Autodesk Inventor part; units mm, degrees
(part 2 of 2)
  line L450 (57.93, 7.062) -> (57.93, 1.062)
  line L451 (63.93, 7.062) -> (57.93, 7.062)
  line L452 (63.93, 1.062) -> (63.93, 7.062)
  line L453 (63.43, 6.562) -> (63.43, 1.562)
  line L454 (63.43, 1.562) -> (58.43, 1.562)
  line L455 (58.43, 1.562) -> (58.43, 6.562)
  line L456 (58.43, 6.562) -> (63.43, 6.562)
  line L457 (57.93, 9.186) -> (63.93, 9.186)
  line L458 (57.93, 15.186) -> (57.93, 9.186)
  line L459 (63.93, 15.186) -> (57.93, 15.186)
  line L460 (63.93, 9.186) -> (63.93, 15.186)
  line L461 (63.43, 14.686) -> (63.43, 9.686)
  line L462 (63.43, 9.686) -> (58.43, 9.686)
  line L463 (58.43, 9.686) -> (58.43, 14.686)
  line L464 (58.43, 14.686) -> (63.43, 14.686)
  line L465 (57.93, 17.31) -> (63.93, 17.31)
  line L466 (57.93, 23.31) -> (57.93, 17.31)
  line L467 (63.93, 23.31) -> (57.93, 23.31)
  line L468 (63.93, 17.31) -> (63.93, 23.31)
  line L469 (63.43, 22.81) -> (63.43, 17.81)
  line L470 (63.43, 17.81) -> (58.43, 17.81)
  line L471 (58.43, 17.81) -> (58.43, 22.81)
  line L472 (58.43, 22.81) -> (63.43, 22.81)
  line L473 (57.93, 25.434) -> (63.93, 25.434)
  line L474 (57.93, 31.434) -> (57.93, 25.434)
  line L475 (63.93, 31.434) -> (57.93, 31.434)
  line L476 (63.93, 25.434) -> (63.93, 31.434)
  line L477 (63.43, 30.934) -> (63.43, 25.934)
  line L478 (63.43, 25.934) -> (58.43, 25.934)
  line L479 (58.43, 25.934) -> (58.43, 30.934)
  line L480 (58.43, 30.934) -> (63.43, 30.934)
  line L481 (57.93, 33.558) -> (63.93, 33.558)
  line L482 (57.93, 39.558) -> (57.93, 33.558)
  line L483 (63.93, 39.558) -> (57.93, 39.558)
  line L484 (63.93, 33.558) -> (63.93, 39.558)
  line L485 (63.43, 39.058) -> (63.43, 34.058)
  line L486 (63.43, 34.058) -> (58.43, 34.058)
  line L487 (58.43, 34.058) -> (58.43, 39.058)
  line L488 (58.43, 39.058) -> (63.43, 39.058)
  line L489 (57.93, 41.682) -> (63.93, 41.682)
  line L490 (57.93, 47.682) -> (57.93, 41.682)
  line L491 (63.93, 47.682) -> (57.93, 47.682)
  line L492 (63.93, 41.682) -> (63.93, 47.682)
  line L493 (63.43, 47.182) -> (63.43, 42.182)
  line L494 (63.43, 42.182) -> (58.43, 42.182)
  line L495 (58.43, 42.182) -> (58.43, 47.182)
  line L496 (58.43, 47.182) -> (63.43, 47.182)
  line L497 (57.93, 49.806) -> (63.93, 49.806)
  line L498 (57.93, 55.806) -> (57.93, 49.806)
  line L499 (63.93, 55.806) -> (57.93, 55.806)
  line L500 (63.93, 49.806) -> (63.93, 55.806)
  line L501 (63.43, 55.306) -> (63.43, 50.306)
  line L502 (63.43, 50.306) -> (58.43, 50.306)
  line L503 (58.43, 50.306) -> (58.43, 55.306)
  line L504 (58.43, 55.306) -> (63.43, 55.306)
  line L505 (57.93, 57.93) -> (63.93, 57.93)
  line L506 (57.93, 63.93) -> (57.93, 57.93)
  line L507 (63.93, 63.93) -> (57.93, 63.93)
  line L508 (63.93, 57.93) -> (63.93, 63.93)
  line L509 (63.43, 63.43) -> (63.43, 58.43)
  line L510 (63.43, 58.43) -> (58.43, 58.43)
  line L511 (58.43, 58.43) -> (58.43, 63.43)
  line L512 (58.43, 63.43) -> (63.43, 63.43)
  point P0 (0, 0)
  dimension "d53" = 0.5
  dimension "d56" = 8.124
  dimension "d59" = 8.124
  constraints: 1024 end point, 4 parallel, 2 horizontal, 2 perpendicular, 1 collinear, 1 vertical, 1010 other
  measures "d53" distance between parallel lines of L1 L5
  measures "d56" distance of L0.start L9.start
  measures "d59" distance of L0.start L65.start
extrude "Extrusion5" add sketch "Sketch2" against normal blind 3.5
body "Solid1"
